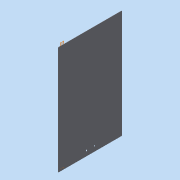
# Autodesk Inventor part: Part23
Saved by Autodesk Inventor 2017 (Build 210142000, 142)
## iProperties
Created: 2018-10-04
Part Number: Part23
Material: Acetal Resin, White
Document SubType Name: Modeling
Designer: mailb
Density: 1.425 g/cm^3
Appearance: Clear
Author: mailb
Autodesk Inventor part; units mm, degrees
ref_plane "YZ Plane" through (0, 0, 0) normal (1, 0, 0) x (0, 1, 0)
ref_plane "XZ Plane" through (0, 0, 0) normal (0, 1, 0) x (-1, 0, 0)
ref_plane "XY Plane" through (0, 0, 0) normal (0, 0, 1) x (1, 0, 0)
ref_plane "Work Plane1" through (48.0967, 298.9917, -302.4032) normal (1, 0, 0) x (0, 1, 0)
sketch "Sketch1" plane through (48.0967, 298.9917, -302.4032) normal (1, 0, 0) x (0, 1, 0)
  circle A0 centre (-276.3, 19.25) radius 3.6
  arc A1 (255.27, -148.59) -> (256.54, -147.32) centre (255.27, -147.32) ccw
  line L0 (256.54, 140.97) -> (256.54, -147.32)
  line L1 (-256.54, 140.97) -> (256.54, 140.97)
  line L2 (-256.54, -147.32) -> (-256.54, 140.97)
  arc A2 (-256.54, -147.32) -> (-255.27, -148.59) centre (-255.27, -147.32) ccw
  line L3 (255.27, -148.59) -> (-255.27, -148.59)
  line L4 (266.7, 140.97) -> (266.7, -154.94)
  line L5 (262.89, -158.75) -> (-262.89, -158.75)
  line L6 (262.89, 158.75) -> (-262.89, 158.75)
  line L7 (-290.7, 29.75) -> (-290.7, 8.75)
  line L8 (266.7, -158.75) -> (-290.7, -158.75)
  line L9 (266.7, 158.75) -> (266.7, -158.75)
  line L10 (-303.2125, 171.2625) -> (-303.2125, -171.2625)
  line L11 (-303.2125, -171.2625) -> (279.2125, -171.2625)
  line L12 (279.2125, -171.2625) -> (279.2125, 171.2625)
  line L13 (279.2125, 171.2625) -> (-303.2125, 171.2625)
  line L14 (-277.69, -21.56) -> (-277.69, -24.16)
  line L15 (-277.69, -24.16) -> (-273.49, -24.16)
  line L16 (-273.49, -24.16) -> (-273.49, -21.56)
  line L17 (-273.49, -21.56) -> (-277.69, -21.56)
  line L18 (-272.25, -25.4) -> (-278.93, -25.4)
  line L19 (-278.93, -25.4) -> (-278.93, -20.32)
  line L20 (-278.93, -20.32) -> (-272.25, -20.32)
  line L21 (-272.25, -20.32) -> (-272.25, -25.4)
  point P0 (-298.9917, 302.4032)
extrude "Extrusion1" add sketch "Sketch1" along normal blind 1 contours L3 A2 L2 L1 L0 A1 | L13 L12 L11 L10 | L18 L19 L20 L21
fillet "Fillet1" radius 3.175 4 edges at (48.5967, -4.2208, -131.1407) (48.5967, -4.2208, -473.6657) (48.5967, 578.2042, -473.6657) (48.5967, 578.2042, -131.1407)
sketch "Sketch2" plane through (49.0967, 298.9917, -302.4032) normal (1, 0, 0) x (0, 0, -1)
  line L0 (21.56, -273.49) -> (24.16, -273.49) projected
  line L1 (21.56, -277.69) -> (21.56, -273.49) projected
  line L2 (24.16, -277.69) -> (21.56, -277.69) projected
  line L3 (24.16, -273.49) -> (24.16, -277.69) projected
  line L4 (24.13, -278.93) -> (21.59, -278.93)
  line L5 (20.32, -277.66) -> (20.32, -273.52)
  line L6 (21.59, -272.25) -> (24.13, -272.25)
  line L7 (25.4, -273.52) -> (25.4, -277.66)
  arc A0 (25.4, -273.52) -> (24.13, -272.25) centre (24.13, -273.52) ccw
  arc A1 (24.13, -278.93) -> (25.4, -277.66) centre (24.13, -277.66) ccw
  arc A2 (20.32, -277.66) -> (21.59, -278.93) centre (21.59, -277.66) ccw
  arc A3 (21.59, -272.25) -> (20.32, -273.52) centre (21.59, -273.52) ccw
  point P0 (-302.4032, -298.9917)
  dimension "d4" = 1.27
  constraints: 8 end point, 8 point on circle, 8 tangent, 4 centre point, 3 equal radius, 3 other
  measures "d4" radius of A0
extrude "Extrusion2" cut sketch "Sketch2" against normal blind 1
body "Solid1"
